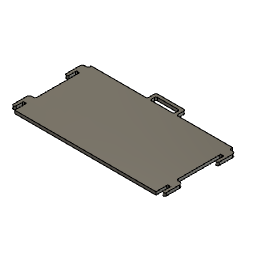
Front_Back_Cut2 (Autodesk Fusion 360 design; units mm, degrees)
Autodesk Fusion 360 part; units mm, degrees
sketch "Sketch1" plane through (0, 0, 0) normal (0, 1, 0) x (1, 0, 0)
  line L0 (0, 0) -> (609.6, 0)
  line L1 (609.6, 0) -> (609.6, -330.2)
  line L2 (609.6, -330.2) -> (0, -330.2)
  line L3 (0, -330.2) -> (0, 0)
  line L4 (609.6, 0) -> (609.6, -12.7) construction
  line L5 (609.6, -12.7) -> (635, -12.7)
  line L6 (635, -12.7) -> (635, -88.9)
  line L7 (609.6, -330.2) -> (609.6, -241.3) construction
  line L8 (609.6, -241.3) -> (635, -241.3)
  line L9 (635, -241.3) -> (635, -317.5)
  line L10 (635, -88.9) -> (622.3, -88.9)
  line L11 (622.3, -88.9) -> (622.3, -50.8)
  line L12 (635, -317.5) -> (622.3, -317.5)
  line L13 (622.3, -317.5) -> (622.3, -279.4)
  line L14 (0, 0) -> (0, -12.7) construction
  line L15 (0, -330.2) -> (0, -241.3) construction
  line L16 (0, -12.7) -> (-25.4, -12.7)
  line L17 (0, -241.3) -> (-25.4, -241.3)
  line L18 (-25.4, -12.7) -> (-25.4, -88.9)
  line L19 (-25.4, -241.3) -> (-25.4, -317.5)
  line L20 (-25.4, -88.9) -> (-12.7, -88.9)
  line L21 (-12.7, -88.9) -> (-12.7, -50.8)
  line L22 (-12.7, -50.8) -> (0, -50.8)
  line L23 (-25.4, -317.5) -> (-12.7, -317.5)
  line L24 (-12.7, -317.5) -> (-12.7, -279.4)
  line L25 (-12.7, -279.4) -> (0, -279.4)
  line L26 (622.3, -50.8) -> (609.6, -50.8)
  line L27 (622.3, -279.4) -> (609.6, -279.5117)
  dimension "d1" = 609.6
  dimension "d18" = 12.7
  dimension "d19" = 25.4
  dimension "d20" = 76.2
  dimension "d21" = 88.9
  dimension "d22" = 25.4
  dimension "d23" = 76.2
  dimension "d24" = 12.7
  dimension "d25" = 38.1
  dimension "d26" = 12.7
  dimension "d27" = 38.1
  dimension "d28" = 12.7
  dimension "d29" = 88.9
  dimension "d30" = 25.4
  dimension "d31" = 25.4
  dimension "d32" = 76.2
  dimension "d33" = 76.2
  dimension "d34" = 38.1
  dimension "d35" = 38.1
  constraint horizontal L0
  constraint vertical L1
  constraint horizontal L2
  constraint vertical L3
  constraint coincident L0.start L3.end
  constraint perpendicular L0 L4
  constraint perpendicular L4 L5
  constraint perpendicular L0 L6
  constraint perpendicular L2 L7
  constraint perpendicular L7 L8
  constraint perpendicular L8 L9
  constraint perpendicular L6 L10
  constraint perpendicular L10 L11
  constraint perpendicular L9 L12
  constraint perpendicular L12 L13
  constraint perpendicular L0 L14
  constraint perpendicular L2 L15
  constraint perpendicular L14 L16
  constraint perpendicular L15 L17
  constraint perpendicular L16 L18
  constraint perpendicular L17 L19
  constraint perpendicular L18 L20
  constraint perpendicular L20 L21
  constraint coincident L3 L22.end
  constraint perpendicular L3 L22
  constraint perpendicular L19 L23
  constraint perpendicular L23 L24
  constraint coincident L15 L25.end
  constraint coincident L1 L26.end
  constraint perpendicular L1 L26
  constraint coincident L1 L27.end
  measures "d1" distance of L0.start L0.end
  measures "d18" distance of L0.end L4.end
  measures "d19" distance of L4.end L5.end
  measures "d20" distance of L5.end L6.end
  measures "d21" distance of L1.end L7.end
  measures "d22" distance of L7.end L8.end
  measures "d23" distance of L8.end L9.end
  measures "d24" distance of L6.end L10.end
  measures "d25" distance of L10.end L11.end
  measures "d26" distance of L9.end L12.end
  measures "d27" distance of L12.end L13.end
  measures "d28" distance of L0.start L14.end
  measures "d29" distance of L2.end L15.end
  measures "d30" distance of L14.end L16.end
  measures "d31" distance of L15.end L17.end
  measures "d32" distance of L16.end L18.end
  measures "d33" distance of L17.end L19.end
  measures "d34" distance of L20.end L21.end
  measures "d35" distance of L23.end L24.end
extrude "Extrude1" add sketch "Sketch1" along normal blind 12.7 in component "Component"
fillet "Fillet1" radius 12.7 4 edges at (635, 6.35, 12.7) (635, 6.35, 241.3) (-25.4, 6.35, 12.7) (-25.4, 6.35, 241.3) in component "Component"
fillet "Fillet2" radius 6.35 2 edges at (-12.7, 6.35, 88.9) (-25.4, 6.35, 88.9) in component "Component"
fillet "Fillet3" radius 6.35 6 edges at (-25.4, 6.35, 317.5) (-12.7, 6.35, 317.5) (622.3, 6.35, 88.9) (635, 6.35, 88.9) (635, 6.35, 317.5) (622.3, 6.35, 317.5) in component "Component"
sketch "Sketch2" plane through (0, 12.7, 0) normal (0, 1, 0) x (-1, 0, 0)
  arc A0 (-622.3, 311.15) -> (-635, 311.15) centre (-628.65, 311.15) ccw
  line L0 (-635, 311.15) -> (-635, 254)
  arc A1 (-635, 254) -> (-622.3, 241.3) centre (-622.3, 254) ccw
  line L1 (-622.3, 241.3) -> (-609.6, 241.3)
  line L2 (-609.6, 241.3) -> (-609.6, 50.8)
  line L3 (-609.6, 50.8) -> (-622.3, 50.8)
  line L4 (-622.3, 50.8) -> (-622.3, 82.55)
  arc A2 (-622.3, 82.55) -> (-635, 82.55) centre (-628.65, 82.55) ccw
  line L5 (-635, 82.55) -> (-635, 25.4)
  arc A3 (-635, 25.4) -> (-622.3, 12.7) centre (-622.3, 25.4) ccw
  line L6 (-622.3, 12.7) -> (-609.6, 12.7)
  line L7 (-609.6, 12.7) -> (-609.6, 0)
  line L8 (-609.6, 0) -> (0, 0)
  line L9 (0, 0) -> (0, 12.7)
  line L10 (0, 12.7) -> (12.7, 12.7)
  arc A4 (12.7, 12.7) -> (25.4, 25.4) centre (12.7, 25.4) ccw
  line L11 (25.4, 25.4) -> (25.4, 82.55)
  arc A5 (25.4, 82.55) -> (19.05, 88.9) centre (19.05, 82.55) ccw
  arc A6 (19.05, 88.9) -> (12.7, 82.55) centre (19.05, 82.55) ccw
  line L12 (12.7, 82.55) -> (12.7, 50.8)
  line L13 (12.7, 50.8) -> (0, 50.8)
  line L14 (0, 50.8) -> (0, 241.3)
  line L15 (0, 241.3) -> (12.7, 241.3)
  arc A7 (12.7, 241.3) -> (25.4, 254) centre (12.7, 254) ccw
  line L16 (25.4, 254) -> (25.4, 311.15)
  arc A8 (25.4, 311.15) -> (19.05, 317.5) centre (19.05, 311.15) ccw
  arc A9 (19.05, 317.5) -> (12.7, 311.15) centre (19.05, 311.15) ccw
  line L17 (12.7, 311.15) -> (12.7, 279.4)
  line L18 (12.7, 279.4) -> (0, 279.4)
  line L19 (0, 279.4) -> (0, 330.2)
  line L20 (0, 330.2) -> (-609.6, 330.2)
  line L21 (-609.6, 330.2) -> (-609.6, 279.5117)
  line L22 (-609.6, 279.5117) -> (-622.3, 279.4)
  line L23 (-622.3, 279.4) -> (-622.3, 311.15)
  line L24 (-304.8, 0) -> (-368.3, 0) construction
  line L25 (-368.3, 0) -> (-368.3, -38.1)
  line L26 (-368.3, -38.1) -> (-241.3, -38.1)
  line L27 (-241.3, -38.1) -> (-241.3, 0)
  line L28 (-304.8, -38.1) -> (-304.8, -12.7) construction
  line L29 (-355.6, 0) -> (-254, 0)
  line L30 (-254, 0) -> (-254, -25.4)
  line L31 (-254, -25.4) -> (-355.6, -25.4)
  line L32 (-355.6, -25.4) -> (-355.6, 0)
  line L33 (-355.6, 0) -> (-254, -25.4) construction
  line L34 (-254, 0) -> (-355.6, -25.4) construction
  point P0 (-304.8, -12.7)
  dimension "d44" = 63.5
  dimension "d45" = 38.1
  dimension "d46" = 127
  dimension "d47" = 25.4
  dimension "d48" = 101.6
  dimension "d49" = 25.4
  constraint midpoint L8 L24.start
  constraint parallel L8 L24
  constraint perpendicular L8 L25
  constraint perpendicular L25 L26
  constraint coincident L8 L27.end
  constraint perpendicular L8 L27
  constraint midpoint L26 L28.start
  constraint perpendicular L26 L28
  constraint horizontal L29
  constraint perpendicular L29 L30
  constraint parallel L29 L31
  constraint parallel L30 L32
  constraint coincident L33 P0
  constraint coincident L34 P0
  constraint coincident P0 L28.end
  measures "d44" distance of L24.start L24.end
  measures "d45" distance of L24.end L25.end
  measures "d46" distance of L25.end L26.end
  measures "d47" distance of L28.start P0
  measures "d48" distance of L30.end L31.end
  measures "d49" distance of L29.end L30.end
extrude "Extrude2" add sketch "Sketch2" against normal up to surface (12.7 mm away) contours L8 L25 L26 L27 L30 L31 L32 in component "Component"
fillet "Fillet4" radius 6.35 7 edges at (241.3, 6.35, 0) (355.6, 6.35, 0) (355.6, 6.35, -25.4) (368.3, 6.35, 0) (254, 6.35, -25.4) (368.3, 6.35, -38.1) (241.3, 6.35, -38.1) in component "Component"
fillet "Fillet5" radius 6.35 1 edges at (254, 6.35, 0) in component "Component"
ref_plane "WorkPlane1" through (609.6, 0, 279.5117) normal (0, 1, 0) x (-1, 0, 0)
sketch "Sketch3" plane through (609.6, 0, 279.5117) normal (0, 1, 0) x (-1, 0, 0)
  line L0 (0, 0) -> (0, 50.6883) construction
  line L1 (-12.7, -0.1117) -> (0, 0) construction
  line L2 (0, 0) -> (-2.2549, 2.2352) construction
  circle A0 centre (-2.2549, 2.2352) radius 3.175
  dimension "d57" = 3.175
  constraint coincident L0.start L1.end
  constraint coincident L0.start A0
  measures "d57" distance of L0.start L2.end
sweep "Sweep1" cut kept parallel profiles "Sketch3" along 1 edges at (609.6, 6.35, 279.5117) section 1 in component "Component"
ref_plane "WorkPlane2" through (622.3, 0, 279.4) normal (0, 1, 0) x (-1, 0, 0)
sketch "Sketch4" plane through (622.3, 0, 279.4) normal (0, 1, 0) x (-1, 0, 0)
  line L0 (0, 0) -> (8.2298, 0.0724) construction
  line L1 (0, 31.75) -> (0, 0) construction
  line L2 (0, 0) -> (2.2352, 2.2549) construction
  circle A0 centre (2.2352, 2.2549) radius 3.175
  dimension "d65" = 3.175
  constraint coincident L0.start L1.end
  constraint coincident L0.start A0
  measures "d65" distance of L0.start L2.end
sweep "Sweep2" cut kept parallel profiles "Sketch4" along 1 edges at (622.3, 6.35, 279.4) section 1 in component "Component"
ref_plane "WorkPlane3" through (622.3, 0, 50.8) normal (0, 1, 0) x (-1, 0, 0)
sketch "Sketch5" plane through (622.3, 0, 50.8) normal (0, 1, 0) x (-1, 0, 0)
  line L0 (0, 0) -> (12.7, 0) construction
  line L1 (0, 31.75) -> (0, 0) construction
  line L2 (0, 0) -> (2.2451, 2.2451) construction
  circle A0 centre (2.2451, 2.2451) radius 3.175
  dimension "d73" = 3.175
  constraint coincident L0.start L1.end
  constraint coincident L0.start A0
  measures "d73" distance of L0.start L2.end
sweep "Sweep3" cut kept parallel profiles "Sketch5" along 1 edges at (622.3, 6.35, 50.8) section 1 in component "Component"
ref_plane "WorkPlane4" through (609.6, 0, 50.8) normal (0, 1, 0) x (-1, 0, 0)
sketch "Sketch6" plane through (609.6, 0, 50.8) normal (0, 1, 0) x (-1, 0, 0)
  line L0 (0, 0) -> (0, 190.5) construction
  line L1 (-8.2099, 0) -> (0, 0) construction
  line L2 (0, 0) -> (-2.2451, 2.2451) construction
  circle A0 centre (-2.2451, 2.2451) radius 3.175
  dimension "d81" = 3.175
  constraint coincident L0.start L1.end
  constraint coincident L0.start A0
  measures "d81" distance of L0.start L2.end
sweep "Sweep4" cut kept parallel profiles "Sketch6" along 1 edges at (609.6, 6.35, 50.8) section 1 in component "Component"
ref_plane "WorkPlane5" through (0, 0, 279.4) normal (0, 1, 0) x (-1, 0, 0)
sketch "Sketch7" plane through (0, 0, 279.4) normal (0, 1, 0) x (-1, 0, 0)
  line L0 (12.7, 0) -> (0, 0) construction
  line L1 (0, 50.8) -> (0, 0) construction
  line L2 (0, 0) -> (2.2451, 2.2451) construction
  circle A0 centre (2.2451, 2.2451) radius 3.175
  dimension "d89" = 3.175
  constraint coincident L0.end L1.end
  constraint coincident L0.end A0
  measures "d89" distance of L0.end L2.end
sweep "Sweep5" cut kept parallel profiles "Sketch7" along 1 edges at (0, 6.35, 279.4) section 1 in component "Component"
ref_plane "WorkPlane6" through (0, 0, 50.8) normal (0, 1, 0) x (-1, 0, 0)
sketch "Sketch8" plane through (0, 0, 50.8) normal (0, 1, 0) x (-1, 0, 0)
  line L0 (12.7, 0) -> (0, 0) construction
  line L1 (0, 190.5) -> (0, 0) construction
  line L2 (0, 0) -> (2.2451, 2.2451) construction
  circle A0 centre (2.2451, 2.2451) radius 3.175
  dimension "d97" = 3.175
  constraint coincident L0.end L1.end
  constraint coincident L0.end A0
  measures "d97" distance of L0.end L2.end
sweep "Sweep6" cut kept parallel profiles "Sketch8" along 1 edges at (0, 6.35, 50.8) section 1 in component "Component"
ref_plane "WorkPlane7" through (-12.7, 0, 50.8) normal (0, 1, 0) x (-1, 0, 0)
sketch "Sketch9" plane through (-12.7, 0, 50.8) normal (0, 1, 0) x (-1, 0, 0)
  line L0 (0, 31.75) -> (0, 0) construction
  line L1 (0, 0) -> (-8.2099, 0) construction
  line L2 (0, 0) -> (-2.2451, 2.2451) construction
  circle A0 centre (-2.2451, 2.2451) radius 3.175
  dimension "d105" = 3.175
  constraint coincident L0.end L1.start
  constraint coincident L0.end A0
  measures "d105" distance of L0.end L2.end
sweep "Sweep7" cut kept parallel profiles "Sketch9" along 1 edges at (-12.7, 6.35, 50.8) section 1 in component "Component"
ref_plane "WorkPlane8" through (-12.7, 0, 279.4) normal (0, 1, 0) x (-1, 0, 0)
sketch "Sketch10" plane through (-12.7, 0, 279.4) normal (0, 1, 0) x (-1, 0, 0)
  line L0 (0, 31.75) -> (0, 0) construction
  line L1 (0, 0) -> (-8.2099, 0) construction
  line L2 (0, 0) -> (-2.2451, 2.2451) construction
  circle A0 centre (-2.2451, 2.2451) radius 3.175
  dimension "d113" = 3.175
  constraint coincident L0.end L1.start
  constraint coincident L0.end A0
  measures "d113" distance of L0.end L2.end
sweep "Sweep8" cut kept parallel profiles "Sketch10" along 1 edges at (-12.7, 6.35, 279.4) section 1 in component "Component"
fillet "Fillet6" radius 6.35 4 edges at (0, 6.35, 241.3) (0, 6.35, 12.7) (609.6, 6.35, 12.7) (609.6, 6.35, 241.3) in component "Component"
component "Component" placed x (1, 0, 0) y (0, 1, 0) z (0, 0, 1) at (0, 0, 0)
equation "d57 = 0.25 in / 2 + 0.00 in"
equation "d65 = 0.25 in / 2 + 0.00 in"
equation "d73 = 0.25 in / 2 + 0.00 in"
equation "d81 = 0.25 in / 2 + 0.00 in"
equation "d89 = 0.25 in / 2 + 0.00 in"
equation "d97 = 0.25 in / 2 + 0.00 in"
equation "d105 = 0.25 in / 2 + 0.00 in"
equation "d113 = 0.25 in / 2 + 0.00 in"
